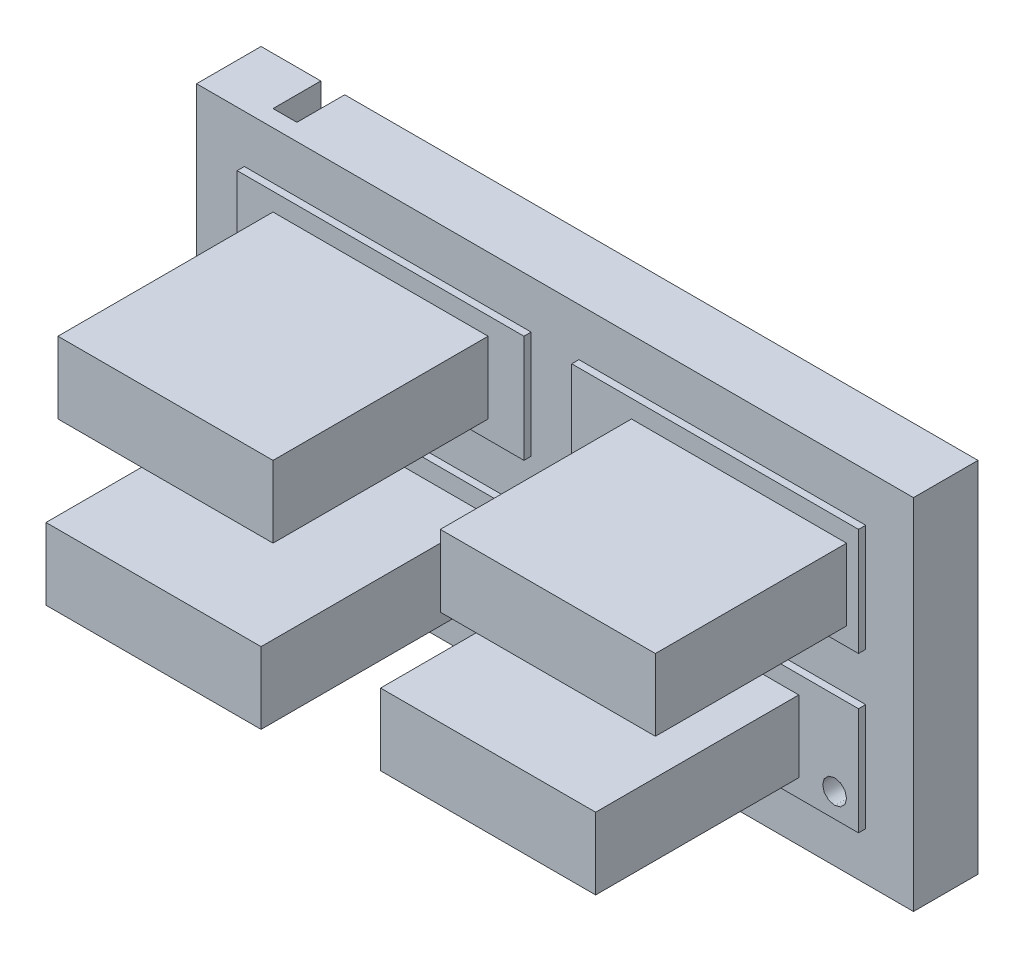
# Autodesk Inventor part: 2
Saved by Autodesk Inventor 2024 (Build 280153000, 153)
## iProperties
Created: 2023-12-11
Part Number: 2
Material: Generisch
Document SubType Name: Modeling
Designer: Luca
Density: 1 g/cm^3
Appearance: Vorgabe
Author: Luca
Autodesk Inventor part; units mm, degrees
ref_plane "YZ Plane" through (0, 0, 0) normal (1, 0, 0) x (0, 1, 0)
ref_plane "XZ Plane" through (0, 0, 0) normal (0, 1, 0) x (-1, 0, 0)
ref_plane "XY Plane" through (0, 0, 0) normal (0, 0, 1) x (1, 0, 0)
sketch "Skizze1" plane through (0, 0, 0) normal (0, 0, 1) x (1, 0, 0)
  line L0 (7309.0058, -3653.1811) -> (7609.0058, -3653.1811)
  line L1 (7609.0058, -3653.1811) -> (7609.0058, -3803.1811)
  line L2 (7609.0058, -3803.1811) -> (7309.0058, -3803.1811)
  line L3 (7309.0058, -3803.1811) -> (7309.0058, -3653.1811)
  point P0 (0, 0)
  dimension "d0" = 300
  dimension "d1" = 150
  constraints: 8 end point, 2 parallel, 1 horizontal, 1 perpendicular
  measures "d0" distance of L1.end L2.end
  measures "d1" distance of L0.end L1.end
extrude "Extrusion1" add sketch "Skizze1" along normal blind 30
sketch "Skizze2" plane through (0, 0, 30) normal (0, 0, 1) x (1, 0, 0)
  line L0 (7309.0058, -3653.1811) -> (7309.0058, -3803.1811) projected
  line L1 (7609.0058, -3803.1811) -> (7609.0058, -3653.1811) projected
  line L2 (7309.0058, -3718.1811) -> (7609.0058, -3718.1811)
  line L3 (7609.0058, -3718.1811) -> (7609.0058, -3738.1811)
  line L4 (7609.0058, -3738.1811) -> (7309.0058, -3738.1811)
  line L5 (7309.0058, -3738.1811) -> (7309.0058, -3718.1811)
  line L6 (7609.0058, -3653.1811) -> (7309.0058, -3653.1811) projected
  point P0 (0, 0)
  dimension "d4" = 20
  dimension "d5" = 65
  constraints: 8 end point, 2 parallel, 2 point on line, 1 horizontal, 1 perpendicular
  measures "d4" distance between parallel lines of L4 L2
  measures "d5" distance between parallel lines of L2 L6
extrude "Extrusion2" cut sketch "Skizze2" against normal blind 3 contours L2 L1 L4 L0
sketch "Skizze3" plane through (0, 0, 30) normal (0, 0, 1) x (1, 0, 0)
  line L0 (7609.0058, -3653.1811) -> (7309.0058, -3653.1811) projected
  line L1 (7309.0058, -3803.1811) -> (7609.0058, -3803.1811) projected
  line L2 (7449.0058, -3653.1811) -> (7469.0058, -3653.1811)
  line L3 (7469.0058, -3653.1811) -> (7469.0058, -3803.1811)
  line L4 (7469.0058, -3803.1811) -> (7449.0058, -3803.1811)
  line L5 (7449.0058, -3803.1811) -> (7449.0058, -3653.1811)
  line L6 (7309.0058, -3653.1811) -> (7309.0058, -3718.1811) projected
  point P0 (0, 0)
  dimension "d8" = 20
  dimension "d9" = 140
  constraints: 8 end point, 2 parallel, 2 point on line, 1 horizontal, 1 perpendicular
  measures "d8" distance of L3.end L4.end
  measures "d9" distance between parallel lines of L6 L5
extrude "Extrusion3" cut sketch "Skizze3" against normal blind 3
sketch "Skizze4" plane through (0, 0, 30) normal (0, 0, 1) x (1, 0, 0)
  line L0 (7609.0058, -3653.1811) -> (7309.0058, -3653.1811) projected
  line L1 (7309.0058, -3803.1811) -> (7609.0058, -3803.1811) projected
  line L2 (7609.0058, -3653.1811) -> (7589.0058, -3653.1811)
  line L3 (7589.0058, -3653.1811) -> (7589.0058, -3803.1811)
  line L4 (7589.0058, -3803.1811) -> (7609.0058, -3803.1811)
  line L5 (7609.0058, -3803.1811) -> (7609.0058, -3653.1811)
  line L6 (7309.0058, -3653.1811) -> (7329.0058, -3653.1811)
  line L7 (7329.0058, -3653.1811) -> (7329.0058, -3803.1811)
  line L8 (7329.0058, -3803.1811) -> (7309.0058, -3803.1811)
  line L9 (7309.0058, -3803.1811) -> (7309.0058, -3653.1811)
  line L10 (7309.0058, -3803.1811) -> (7609.0058, -3803.1811)
  line L11 (7609.0058, -3803.1811) -> (7609.0058, -3783.1811)
  line L12 (7609.0058, -3783.1811) -> (7309.0058, -3783.1811)
  line L13 (7309.0058, -3783.1811) -> (7309.0058, -3803.1811)
  line L14 (7609.0058, -3653.1811) -> (7309.0058, -3653.1811)
  line L15 (7309.0058, -3653.1811) -> (7309.0058, -3673.1811)
  line L16 (7309.0058, -3673.1811) -> (7609.0058, -3673.1811)
  line L17 (7609.0058, -3673.1811) -> (7609.0058, -3653.1811)
  point P0 (0, 0)
  point P1 (7589.0058, -3783.1811)
  point P2 (7329.0058, -3783.1811)
  point P3 (7329.0058, -3673.1811)
  point P4 (7589.0058, -3673.1811)
  dimension "d12" = 20
  dimension "d13" = 20
  dimension "d14" = 20
  dimension "d15" = 20
  constraints: 32 end point, 8 parallel, 5 point on line, 4 horizontal, 4 perpendicular
  measures "d12" distance of L4.end L3.end
  measures "d13" distance of L7.end L8.end
  measures "d14" distance of L11.end L10.end
  measures "d15" distance of L15.end L14.end
extrude "Extrusion4" cut sketch "Skizze4" against normal blind 3 contours L5 L16 L3 L0 | L3 L16 L7 L0 | L5 L12 L3 L16 | L7 L16 L9 L0 | L5 L1 L3 L12 | L7 L12 L9 L16 | L3 L1 L7 L12 | L7 L1 L9 L12
sketch "Skizze5" plane through (0, 0, 30) normal (0, 0, 1) x (1, 0, 0)
  line L0 (7344.0058, -3680.6811) -> (7434.0058, -3680.6811)
  line L1 (7434.0058, -3680.6811) -> (7434.0058, -3710.6811)
  line L2 (7434.0058, -3710.6811) -> (7344.0058, -3710.6811)
  line L3 (7344.0058, -3710.6811) -> (7344.0058, -3680.6811)
  line L4 (7449.0058, -3673.1811) -> (7329.0058, -3673.1811) projected
  line L5 (7329.0058, -3673.1811) -> (7329.0058, -3718.1811) projected
  line L6 (7344.0058, -3745.6811) -> (7434.0058, -3745.6811)
  line L7 (7434.0058, -3745.6811) -> (7434.0058, -3775.6811)
  line L8 (7434.0058, -3775.6811) -> (7344.0058, -3775.6811)
  line L9 (7344.0058, -3775.6811) -> (7344.0058, -3745.6811)
  line L10 (7449.0058, -3738.1811) -> (7329.0058, -3738.1811) projected
  line L11 (7449.0058, -3783.1811) -> (7449.0058, -3738.1811) projected
  line L12 (7474.0058, -3745.6811) -> (7564.0058, -3745.6811)
  line L13 (7564.0058, -3745.6811) -> (7564.0058, -3775.6811)
  line L14 (7564.0058, -3775.6811) -> (7474.0058, -3775.6811)
  line L15 (7474.0058, -3775.6811) -> (7474.0058, -3745.6811)
  line L16 (7589.0058, -3738.1811) -> (7469.0058, -3738.1811) projected
  line L17 (7469.0058, -3738.1811) -> (7469.0058, -3783.1811) projected
  line L18 (7494.0058, -3680.6811) -> (7584.0058, -3680.6811)
  line L19 (7584.0058, -3680.6811) -> (7584.0058, -3710.6811)
  line L20 (7584.0058, -3710.6811) -> (7494.0058, -3710.6811)
  line L21 (7494.0058, -3710.6811) -> (7494.0058, -3680.6811)
  line L22 (7589.0058, -3673.1811) -> (7469.0058, -3673.1811) projected
  line L23 (7589.0058, -3718.1811) -> (7589.0058, -3673.1811) projected
  line L24 (7609.0058, -3803.1811) -> (7309.0058, -3803.1811) projected
  line L25 (7309.0058, -3803.1811) -> (7309.0058, -3653.1811) projected
  line L26 (7609.0058, -3653.1811) -> (7609.0058, -3803.1811) projected
  line L27 (7309.0058, -3653.1811) -> (7609.0058, -3653.1811) projected
  point P0 (0, 0)
  point P1 (7329.0058, -3695.6811)
  point P2 (7564.0058, -3760.6811)
  dimension "d18" = 90
  dimension "d19" = 30
  dimension "d20" = 7.5
  dimension "d21" = 15
  dimension "d22" = 90
  dimension "d23" = 30
  dimension "d24" = 7.5
  dimension "d25" = 15
  dimension "d26" = 90
  dimension "d27" = 30
  dimension "d28" = 7.5
  dimension "d29" = 5
  dimension "d30" = 90
  dimension "d31" = 30
  dimension "d32" = 7.5
  dimension "d33" = 5
  dimension "d58" = 27.5
  dimension "d59" = 35
  dimension "d60" = 35
  dimension "d61" = 45
  dimension "d62" = 27.5
  dimension "d63" = 25
  dimension "d64" = 27.5
  constraints: 32 end point, 8 parallel, 4 horizontal, 4 perpendicular, 2 midpoint
  measures "d18" distance of L1.end L2.end
  measures "d19" distance of L0.end L1.end
  measures "d20" distance between parallel lines of L4 L0
  measures "d21" distance from line of point (7329.006, -3695.681) L3
  measures "d22" distance of L7.end L8.end
  measures "d23" distance of L6.end L7.end
  measures "d24" distance between parallel lines of L6 L10
  measures "d25" distance between parallel lines of L11 L7
  measures "d26" distance of L13.end L14.end
  measures "d27" distance of L12.end L13.end
  measures "d28" distance between parallel lines of L16 L12
  measures "d29" distance between parallel lines of L17 L15
  measures "d30" distance of L19.end L20.end
  measures "d31" distance of L18.end L19.end
  measures "d32" distance between parallel lines of L22 L18
  measures "d33" distance between parallel lines of L23 L19
  measures "d58" distance between parallel lines of L24 L8
  measures "d59" distance between parallel lines of L25 L9
  measures "d60" distance between parallel lines of L6 L2
  measures "d61" distance from line of L26 point (7564.006, -3760.681)
  measures "d62" distance between parallel lines of L24 L14
  measures "d63" distance between parallel lines of L26 L19
  measures "d64" distance between parallel lines of L27 L18
extrude "Extrusion5" add sketch "Skizze5" along normal blind 90 contours L0 L1 L2 L3
extrude "Extrusion6" add sketch "Skizze5" along normal blind 80 contours L18 L19 L20 L21
extrude "Extrusion7" add sketch "Skizze5" along normal blind 95 contours L6 L7 L8 L9
extrude "Extrusion8" add sketch "Skizze5" along normal blind 85 contours L12 L13 L14 L15
sketch "Skizze6" plane through (0, 0, 0) normal (0, 0, -1) x (-1, 0, 0)
  line L0 (-7599.0058, -3663.1811) -> (-7319.0058, -3663.1811)
  line L1 (-7319.0058, -3663.1811) -> (-7319.0058, -3793.1811)
  line L2 (-7319.0058, -3793.1811) -> (-7599.0058, -3793.1811)
  line L3 (-7599.0058, -3793.1811) -> (-7599.0058, -3663.1811)
  line L4 (-7609.0058, -3653.1811) -> (-7309.0058, -3653.1811) projected
  line L5 (-7609.0058, -3803.1811) -> (-7609.0058, -3653.1811) projected
  line L6 (-7344.0058, -3653.1811) -> (-7334.0058, -3653.1811)
  line L7 (-7334.0058, -3653.1811) -> (-7334.0058, -3663.1811)
  line L8 (-7334.0058, -3663.1811) -> (-7344.0058, -3663.1811)
  line L9 (-7344.0058, -3663.1811) -> (-7344.0058, -3653.1811)
  line L10 (-7309.0058, -3653.1811) -> (-7309.0058, -3803.1811) projected
  point P0 (0, 0)
  point P1 (-7334.0058, -3658.1811)
  dimension "d42" = 280
  dimension "d43" = 130
  dimension "d44" = 10
  dimension "d45" = 10
  dimension "d46" = 10
  dimension "d47" = 25
  constraints: 16 end point, 4 parallel, 2 horizontal, 2 perpendicular, 2 point on line, 1 midpoint
  measures "d42" distance of L1.end L2.end
  measures "d43" distance of L0.end L1.end
  measures "d44" distance between parallel lines of L4 L0
  measures "d45" distance between parallel lines of L5 L3
  measures "d46" distance of L7.end L8.end
  measures "d47" distance from line of L10 point (-7334.006, -3658.181)
extrude "Extrusion9" cut sketch "Skizze6" against normal blind 20
sketch "Skizze7" plane through (0, 0, 30) normal (0, 0, 1) x (1, 0, 0)
  circle A0 centre (7479.0058, -3708.1811) radius 5
  circle A1 centre (7579.0058, -3773.1811) radius 5
  line L0 (7469.0058, -3673.1811) -> (7469.0058, -3718.1811) projected
  line L1 (7469.0058, -3718.1811) -> (7589.0058, -3718.1811) projected
  line L2 (7589.0058, -3783.1811) -> (7589.0058, -3738.1811) projected
  line L3 (7469.0058, -3783.1811) -> (7589.0058, -3783.1811) projected
  point P0 (0, 0)
  dimension "d50" = 10
  dimension "d51" = 10
  dimension "d52" = 10
  dimension "d53" = 10
  dimension "d54" = 10
  dimension "d55" = 10
  constraints: 2 centre point
  measures "d50" diameter of A0
  measures "d51" diameter of A1
  measures "d52" distance from line of L0 A0.centre
  measures "d53" distance from line of L1 A0.centre
  measures "d54" distance from line of L2 A1.centre
  measures "d55" distance from line of L3 A1.centre
extrude "Extrusion10" cut sketch "Skizze7" against normal through all
sketch "Skizze8" plane through (0, 0, 20) normal (0, 0, -1) x (-1, 0, 0)
  line L0 (-7349.0058, -3685.6811) -> (-7429.0058, -3685.6811)
  line L1 (-7429.0058, -3685.6811) -> (-7429.0058, -3705.6811)
  line L2 (-7429.0058, -3705.6811) -> (-7349.0058, -3705.6811)
  line L3 (-7349.0058, -3705.6811) -> (-7349.0058, -3685.6811)
  line L4 (-7609.0058, -3653.1811) -> (-7344.0058, -3653.1811) projected
  line L5 (-7309.0058, -3653.1811) -> (-7309.0058, -3803.1811) projected
  point P0 (0, 0)
  dimension "d65" = 80
  dimension "d66" = 20
  dimension "d67" = 32.5
  dimension "d68" = 40
  constraints: 8 end point, 2 parallel, 1 horizontal, 1 perpendicular
  measures "d65" distance of L2.end L1.end
  measures "d66" distance of L1.end L0.end
  measures "d67" distance between parallel lines of L0 L4
  measures "d68" distance between parallel lines of L5 L3
